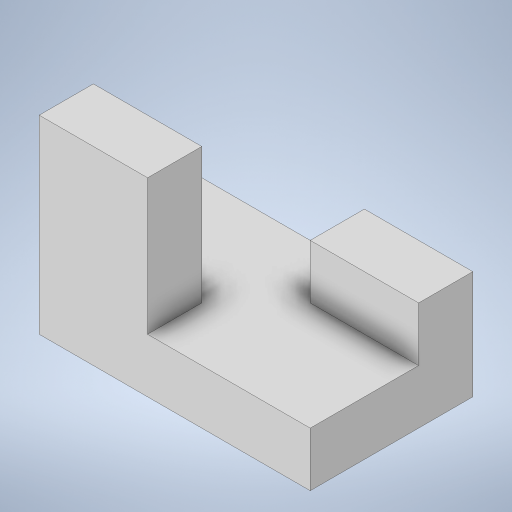
# Autodesk Inventor part: BT004_Formstück
Saved by Autodesk Inventor 2023 (Build 270158000, 158)
## iProperties
Created: 2022-04-26
Part Number: BT004_Formstück
Material: Generic
Document SubType Name: Modeling
Designer: Altar
Density: 1 g/cm^3
Appearance: Default
Author: Altar
Autodesk Inventor part; units mm, degrees
ref_plane "YZ Plane" through (0, 0, 0) normal (1, 0, 0) x (0, 1, 0)
ref_plane "XZ Plane" through (0, 0, 0) normal (0, 1, 0) x (-1, 0, 0)
ref_plane "XY Plane" through (0, 0, 0) normal (0, 0, 1) x (1, 0, 0)
sketch "Sketch1" plane through (0, 0, 0) normal (1, 0, 0) x (0, 1, 0)
  line L0 (-2.71, -15.0951) -> (7.29, -15.0951)
  line L1 (7.29, -15.0951) -> (7.29, 34.9049)
  line L2 (7.29, 34.9049) -> (-2.71, 34.9049)
  line L3 (-2.71, 34.9049) -> (-2.71, -15.0951)
  point P0 (0, 0)
  dimension "d0" = 50
  dimension "d1" = 10
  constraints: 8 end point, 3 perpendicular, 1 horizontal
  measures "d0" distance of L0.end L1.end
  measures "d1" distance of L0.start L0.end
extrude "Extrusion1" add sketch "Sketch1" along normal blind 30
sketch "Sketch2" plane through (0, 0, 0) normal (1, 0, 0) x (0, 1, 0)
  line L0 (7.29, -15.0951) -> (7.29, 34.9049) projected
  line L1 (7.29, -15.0951) -> (32.29, -15.0951)
  line L2 (32.29, -15.0951) -> (32.29, 4.9049)
  line L3 (32.29, 4.9049) -> (7.29, 4.9049)
  point P0 (0, 0)
  dimension "d4" = 25
  dimension "d5" = 20
  constraints: 6 end point, 2 perpendicular, 1 horizontal, 1 point on line
  measures "d4" distance of L0.start L1.end
  measures "d5" distance of L1.end L2.end
extrude "Extrusion2" add sketch "Sketch2" along normal blind 10
sketch "Sketch3" plane through (30, 0, 0) normal (1, 0, 0) x (0, 0, -1)
  line L0 (-34.9049, 7.29) -> (-34.9049, -2.71) projected
  line L1 (-34.9049, 7.29) -> (-34.9049, 17.29)
  line L2 (-34.9049, 17.29) -> (-14.9049, 17.29)
  line L3 (-14.9049, 17.29) -> (-14.9049, 7.29)
  line L4 (15.0951, 7.29) -> (-34.9049, 7.29) projected
  line L5 (-14.9049, 7.29) -> (-34.9049, 7.29)
  point P0 (0, 0)
  dimension "d8" = 20
  dimension "d9" = 10
  constraints: 8 end point, 2 perpendicular, 1 collinear, 1 vertical
  measures "d8" distance of L1.end L2.end
  measures "d9" distance of L0.start L1.end
extrude "Extrusion3" add sketch "Sketch3" against normal blind 10
body "Solid1"
